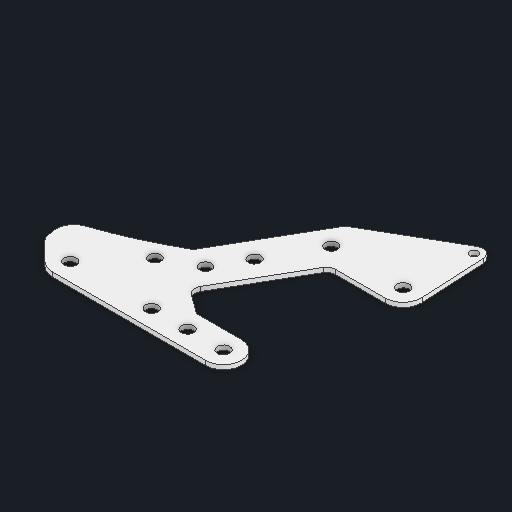
# Autodesk Inventor part: Funnel Gusset Back Improved V2
Saved by Autodesk Inventor 2025.1 (Build 291241000, 241)
## iProperties
Created: 2024-10-23
Part Number: Funnel Gusset Back Improved V2
Material: Acetal Resin, White
Document SubType Name: Modeling
Designer: avere
Density: 1.425 g/cm^3
Appearance: Smooth - White
d2: 0.172 in
d3: 0.172 in
d13: 0.250 in
d59: 10.000 in
Author: avere
Autodesk Inventor part; units mm, degrees
ref_plane "YZ Plane" through (0, 0, 0) normal (1, 0, 0) x (0, 1, 0)
ref_plane "XZ Plane" through (0, 0, 0) normal (0, 1, 0) x (-1, 0, 0)
ref_plane "XY Plane" through (0, 0, 0) normal (0, 0, 1) x (1, 0, 0)
sketch "main" plane through (0, 0, 0) normal (0, 0, 1) x (1, 0, 0)
  circle A0 centre (36.4896, 64.2776) radius 2.1844
  line L0 (36.4904, 70.6276) -> (-17.6528, 70.6344)
  circle A1 centre (7.7473, 64.2844) radius 2.1844
  line L1 (-17.6416, 57.9344) -> (-1.7768, 57.9386)
  arc A2 (-17.6528, 70.6344) -> (-17.6416, 57.9344) centre (-17.6528, 64.2844) ccw
  circle A3 centre (-17.6528, 64.2844) radius 2.1844
  arc A4 (40.98, 68.7674) -> (36.4904, 70.6276) centre (36.4896, 64.2776) ccw
  line L2 (40.98, 68.7674) -> (49.8505, 68.7674) construction
  circle A5 centre (-4.9416, 13.4844) radius 2.1844
  circle A6 centre (-4.9528, 64.287) radius 2.1844
  point P0 (10.5119, 26.5593)
  point P1 (34.4277, 26.6577)
  dimension "d2" = 4.3688
  dimension "d3" = 4.3688
  dimension "d13" = 6.35
  dimension "d78" = 4.3688
  measures "d2" diameter of A0
  measures "d3" diameter of A1
  measures "d13" radius of A2
  measures "d78" diameter of A6
sketch "mogo" plane through (0, 0, 0) normal (0, 0, 1) x (1, 0, 0)
  line L0 (-61.3822, 498.7735) -> (65.6178, 572.097)
  line L1 (65.6178, 572.097) -> (192.6178, 498.7735)
  line L2 (192.6178, 498.7735) -> (192.6178, 352.1265)
  line L3 (192.6178, 352.1265) -> (65.6178, 278.803)
  line L4 (65.6178, 278.803) -> (-61.3822, 352.1265)
  line L5 (-61.3822, 352.1265) -> (-61.3822, 498.7735)
  point P0 (65.6178, 425.45)
  point P1 (65.6178, 425.45)
  dimension "d59" = 254
  measures "d59" distance between parallel lines of L2 L5
sketch "Sketch1" plane through (0, 0, 0) normal (0, 1, 0) x (-1, 0, 0)
  line L0 (58.6337, 4.471) -> (65.1127, -2.0089)
  arc A0 (65.935, -3.4345) -> (65.1127, -2.0089) centre (62.8675, -4.2538) ccw
  circle A1 centre (22.3424, -33.2913) radius 2.1844
  arc A2 (66.587, -6.4669) -> (65.935, -3.4345) centre (35.461, -11.5736) ccw
  arc A3 (62.3569, -13.5096) -> (66.587, -6.4669) centre (60.3208, -7.4949) ccw
  line L1 (31.7488, -5.4171) -> (31.751, 4.6095) projected
  arc A4 (62.3569, -13.5096) -> (36.0563, -25.4131) centre (109.3798, -152.4131) ccw
  line L2 (36.0563, -25.4131) -> (17.2601, -57.9692)
  line L3 (7.6511, -42.8625) -> (23.5038, -15.4048)
  line L4 (49.7771, -4.633) -> (49.6408, -4.4967)
  line L5 (4.9014, -44.45) -> (-12.7, -44.45)
  line L6 (-17.8837, -73.9061) -> (-19.0418, -51.1224)
  line L7 (14.9358, -60.2934) -> (-13.1253, -76.4945)
  circle A5 centre (-12.7, -50.8) radius 2.1844
  arc A6 (-12.7, -44.45) -> (-19.0418, -51.1224) centre (-12.7, -50.8) ccw
  arc A7 (-17.8837, -73.9061) -> (-13.1253, -76.4945) centre (-14.7128, -73.7449) ccw
  circle A8 centre (-14.7128, -73.7449) radius 1.4693
  arc A9 (14.9358, -60.2934) -> (17.2601, -57.9692) centre (11.7608, -54.7942) ccw
  circle A10 centre (28.6924, -22.2928) radius 2.0955
  line L8 (22.62, -11.2484) -> (15.8746, -6.349)
  arc A11 (23.5038, -15.4048) -> (22.62, -11.2484) centre (20.7541, -13.8173) ccw
  circle A12 centre (40.2193, -15.9401) radius 2.0955
  arc A13 (4.9014, -44.45) -> (7.6511, -42.8625) centre (4.9014, -41.275) ccw
  circle A14 centre (54.1423, -0.0179) radius 2.1844
  line L9 (54.1445, 6.3321) -> (0.0013, 6.35)
  circle A15 centre (25.4, -0.0052) radius 2.1844
  line L10 (0.0098, -6.35) -> (15.8746, -6.349)
  arc A16 (0.0013, 6.35) -> (0.0098, -6.35) centre (0, 0) ccw
  circle A17 centre (0, 0) radius 2.1844
  arc A18 (58.6337, 4.471) -> (54.1445, 6.3321) centre (54.1423, -0.0179) ccw
  line L11 (58.6337, 4.471) -> (67.5042, 4.4692) construction
  circle A19 centre (12.7007, -50.8026) radius 2.1844
  circle A20 centre (12.7, 0) radius 2.1844
  point P0 (0, 0)
  point P1 (65.6981, -2.5943)
  point P2 (58.6337, 4.471)
  point P3 (-17.6202, -79.0897)
  point P4 (16.4093, -59.4427)
  point P5 (15.8746, -6.349)
  dimension "d41" = 3.175
  dimension "d54" = 4.3688
  dimension "d60" = 6.35
  dimension "d64" = 15.875
  dimension "d65" = 4.3688
  dimension "d66" = 12.7
  dimension "d67" = 3.175
  dimension "d68" = 6.35
  dimension "d69" = 4.191
  dimension "d70" = 7.9375
  dimension "d71" = 12.7
  dimension "d72" = 7.9375
  dimension "d75" = 3.175
  dimension "d76" = 4.191
  dimension "d77" = 3.175
  constraints: 18 point on circle, 16 end point, 14 centre point, 11 tangent, 5 point on line, 2 coincident, 1 horizontal, 9 other
  measures "d41" radius of A0
  measures "d54" diameter of A1
  measures "d60" radius of A3
  measures "d64" distance between parallel lines of L2 L3
  measures "d65" diameter of A5
  measures "d66" diameter of A6
  measures "d67" radius of A7
  measures "d68" radius of A9
  measures "d69" diameter of A10
  measures "d70" distance from line of L3 A10.centre
  measures "d71" distance of A1.centre A10.centre
  measures "d72" distance from line of L3 A1.centre
  measures "d75" radius of A11
  measures "d76" diameter of A12
  measures "d77" radius of A13
extrude "Extrusion1" add sketch "Sketch1" along normal blind 1.5875
body "Solid1"
